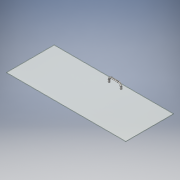
# Autodesk Inventor part: doorLeft
Saved by Autodesk Inventor 2019 (Build 230136000, 136)
## iProperties
Created: 2018-09-21
Part Number: doorLeft
Material: Glass
Document SubType Name: Modeling
Designer: wade
Density: 2.18 g/cm^3
Appearance: Clear
Author: wade
Autodesk Inventor part; units mm, degrees
ref_plane "YZ Plane" through (0, 0, 0) normal (1, 0, 0) x (0, 1, 0)
sketch "Sketch1" plane through (0, 0, 0) normal (0, 1, 0) x (-1, 0, 0)
  line L0 (0, 0) -> (2500, 0)
  line L1 (2500, 0) -> (2500, -1000)
  line L2 (2500, -1000) -> (0, -1000)
  line L3 (0, -1000) -> (0, 0)
  dimension "d0" = 2500
  dimension "d1" = 1000
  constraints: 8 end point, 2 parallel, 1 horizontal, 1 perpendicular
  measures "d0" distance of L1.end L2.end
  measures "d1" distance of L0.end L1.end
extrude "Extrusion1" add sketch "Sketch1" along normal blind 10
sketch "Sketch2" plane through (0, 10, 0) normal (0, 1, 0) x (1, 0, 0)
  line L0 (-2500, 0) -> (0, 0) projected
  line L1 (0, 0) -> (0, 1000) projected
  line L2 (0, 1000) -> (-2500, 1000) projected
  line L3 (-2500, 1000) -> (-2500, 0) projected
  circle A0 centre (-1250, 900) radius 17.5
  dimension "d4" = 35
  dimension "d5" = 100
  dimension "d6" = 1250
  constraints: 1 centre point
  measures "d4" diameter of A0
  measures "d5" distance from line of L2 A0.centre
  measures "d6" distance from line of L1 A0.centre
ref_plane "Work Plane1" through (0, 0, -900) normal (0, 0, -1) x (-1, 0, 0)
sketch "Sketch3" plane through (0, 0, -900) normal (0, 0, -1) x (-1, 0, 0)
  line L0 (1000, 10) -> (1000, 60)
  line L1 (1050, 110) -> (1200, 110)
  line L2 (1250, 60) -> (1250, 10)
  arc A0 (1050, 110) -> (1000, 60) centre (1050, 60) ccw
  arc A1 (1250, 60) -> (1200, 110) centre (1200, 60) ccw
  point P0 (0, 0)
  point P1 (1000, 110)
  point P2 (1250, 110)
  dimension "d8" = 250
  dimension "d9" = 100
  dimension "d10" = 50
  dimension "d11" = 250
  constraints: 6 end point, 4 point on circle, 4 point on line, 4 tangent, 2 centre point, 2 parallel, 1 equal radius, 1 horizontal
  measures "d8" distance of point (1000, 110) point (1250, 110)
  measures "d9" distance of L0.start point (1000, 110)
  measures "d10" radius of A0
  measures "d11" distance between parallel lines of L2 L0
sweep "Sweep1" add profiles "Sketch2" path "Sketch3" contours A0
ref_plane "Work Plane2" through (0, 10, 0) normal (0, 1, 0) x (1, 0, 0)
split body "Split1" result two bodies by plane through (0, 10, 0) normal (0, 1, 0) first body at (-1150, 93.2201, -902.727)
body "Solid2"
body "Solid3"
